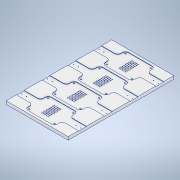
# Autodesk Inventor part: Tamale Assembly Plate
Saved by Autodesk Inventor 2022 (Build 260153000, 153)
## iProperties
Created: 2021-07-16
Part Number: Tamale Assembly Plate
Material: Aluminum 6061
Document SubType Name: Modeling
Designer: Caleb
Density: 2.7 g/cm^3
Appearance: Aluminum - Flat
Author: Caleb
Autodesk Inventor part; units mm, degrees
ref_plane "YZ Plane" through (0, 0, 0) normal (1, 0, 0) x (0, 1, 0)
ref_plane "XZ Plane" through (0, 0, 0) normal (0, 1, 0) x (-1, 0, 0)
ref_plane "XY Plane" through (0, 0, 0) normal (0, 0, 1) x (1, 0, 0)
sketch "Sketch1" plane through (0, 0, 0) normal (0, 1, 0) x (-1, 0, 0)
  line L0 (-63.5, 107.95) -> (63.5, 107.95)
  line L1 (63.5, 107.95) -> (63.5, -107.95)
  line L2 (63.5, -107.95) -> (-63.5, -107.95)
  line L3 (-63.5, -107.95) -> (-63.5, 107.95)
  line L4 (-63.5, 107.95) -> (63.5, -107.95) construction
  line L5 (63.5, 107.95) -> (-63.5, -107.95) construction
  point P0 (0, 0)
  dimension "d0" = 215.9
  dimension "d1" = 127
  constraints: 12 end point, 2 midpoint, 2 parallel, 1 horizontal, 1 perpendicular
  measures "d0" distance of L0.end L1.end
  measures "d1" distance of L1.end L2.end
extrude "Extrusion1" add sketch "Sketch1" along normal blind 6.35
sketch "Sketch2" plane through (0, 6.35, 0) normal (0, 1, 0) x (1, 0, 0)
  line L0 (23.8125, -102.87) -> (-23.8125, -102.87)
  line L1 (-30.1625, -96.52) -> (-30.1625, -93.345)
  line L2 (-23.8125, -55.245) -> (23.8125, -55.245)
  line L3 (30.1625, -93.345) -> (30.1625, -96.52)
  line L4 (30.1625, -102.87) -> (-30.1625, -55.245) construction
  line L5 (-30.1625, -102.87) -> (30.1625, -55.245) construction
  line L6 (-63.5, 107.95) -> (-63.5, -107.95) projected
  line L7 (-36.5125, -86.995) -> (-63.5, -86.995)
  line L8 (-63.5, -86.995) -> (-63.5, -71.12)
  line L9 (-63.5, -71.12) -> (-36.5125, -71.12)
  line L10 (63.5, -107.95) -> (63.5, 107.95) projected
  line L11 (36.5125, -71.12) -> (63.5, -71.12)
  line L12 (63.5, -71.12) -> (63.5, -86.995)
  line L13 (63.5, -86.995) -> (36.5125, -86.995)
  arc A0 (-30.1625, -96.52) -> (-23.8125, -102.87) centre (-23.8125, -96.52) ccw
  arc A1 (23.8125, -102.87) -> (30.1625, -96.52) centre (23.8125, -96.52) ccw
  arc A2 (-30.1625, -93.345) -> (-36.5125, -86.995) centre (-36.5125, -93.345) ccw
  arc A3 (36.5125, -86.995) -> (30.1625, -93.345) centre (36.5125, -93.345) ccw
  line L14 (-30.1625, -64.77) -> (-30.1625, -61.595)
  line L15 (30.1625, -64.77) -> (30.1625, -61.595)
  arc A4 (-36.5125, -71.12) -> (-30.1625, -64.77) centre (-36.5125, -64.77) ccw
  arc A5 (30.1625, -64.77) -> (36.5125, -71.12) centre (36.5125, -64.77) ccw
  arc A6 (30.1625, -61.595) -> (23.8125, -55.245) centre (23.8125, -61.595) ccw
  arc A7 (-23.8125, -55.245) -> (-30.1625, -61.595) centre (-23.8125, -61.595) ccw
  arc A8 (30.1625, -8.89) -> (23.8125, -2.54) centre (23.8125, -8.89) ccw
  line L16 (30.1625, -12.065) -> (30.1625, -8.89)
  line L17 (36.5125, -18.415) -> (63.5, -18.415)
  arc A9 (30.1625, -12.065) -> (36.5125, -18.415) centre (36.5125, -12.065) ccw
  line L18 (63.5, -18.415) -> (63.5, -34.29)
  line L19 (63.5, -34.29) -> (36.5125, -34.29)
  line L20 (-23.8125, -2.54) -> (23.8125, -2.54)
  line L21 (30.1625, -40.64) -> (30.1625, -43.815)
  arc A10 (23.8125, -50.165) -> (30.1625, -43.815) centre (23.8125, -43.815) ccw
  line L22 (-30.1625, -43.815) -> (-30.1625, -40.64)
  line L23 (23.8125, -50.165) -> (-23.8125, -50.165)
  line L24 (-30.1625, -50.165) -> (30.1625, -2.54) construction
  line L25 (30.1625, -50.165) -> (-30.1625, -2.54) construction
  arc A11 (36.5125, -34.29) -> (30.1625, -40.64) centre (36.5125, -40.64) ccw
  line L26 (-36.5125, -34.29) -> (-63.5, -34.29)
  line L27 (-63.5, -34.29) -> (-63.5, -18.415)
  line L28 (-63.5, -18.415) -> (-36.5125, -18.415)
  arc A12 (-23.8125, -2.54) -> (-30.1625, -8.89) centre (-23.8125, -8.89) ccw
  line L29 (-30.1625, -12.065) -> (-30.1625, -8.89)
  arc A13 (-36.5125, -18.415) -> (-30.1625, -12.065) centre (-36.5125, -12.065) ccw
  arc A14 (-30.1625, -43.815) -> (-23.8125, -50.165) centre (-23.8125, -43.815) ccw
  arc A15 (-30.1625, -40.64) -> (-36.5125, -34.29) centre (-36.5125, -40.64) ccw
  arc A16 (30.1625, 43.815) -> (23.8125, 50.165) centre (23.8125, 43.815) ccw
  line L30 (30.1625, 40.64) -> (30.1625, 43.815)
  line L31 (36.5125, 34.29) -> (63.5, 34.29)
  arc A17 (30.1625, 40.64) -> (36.5125, 34.29) centre (36.5125, 40.64) ccw
  line L32 (63.5, 34.29) -> (63.5, 18.415)
  line L33 (63.5, 18.415) -> (36.5125, 18.415)
  line L34 (-23.8125, 50.165) -> (23.8125, 50.165)
  line L35 (30.1625, 12.065) -> (30.1625, 8.89)
  arc A18 (23.8125, 2.54) -> (30.1625, 8.89) centre (23.8125, 8.89) ccw
  line L36 (-30.1625, 8.89) -> (-30.1625, 12.065)
  line L37 (23.8125, 2.54) -> (-23.8125, 2.54)
  line L38 (-30.1625, 2.54) -> (30.1625, 50.165) construction
  line L39 (30.1625, 2.54) -> (-30.1625, 50.165) construction
  arc A19 (36.5125, 18.415) -> (30.1625, 12.065) centre (36.5125, 12.065) ccw
  line L40 (-36.5125, 18.415) -> (-63.5, 18.415)
  line L41 (-63.5, 18.415) -> (-63.5, 34.29)
  line L42 (-63.5, 34.29) -> (-36.5125, 34.29)
  arc A20 (-23.8125, 50.165) -> (-30.1625, 43.815) centre (-23.8125, 43.815) ccw
  line L43 (-30.1625, 40.64) -> (-30.1625, 43.815)
  arc A21 (-36.5125, 34.29) -> (-30.1625, 40.64) centre (-36.5125, 40.64) ccw
  arc A22 (-30.1625, 8.89) -> (-23.8125, 2.54) centre (-23.8125, 8.89) ccw
  arc A23 (-30.1625, 12.065) -> (-36.5125, 18.415) centre (-36.5125, 12.065) ccw
  arc A24 (30.1625, 96.52) -> (23.8125, 102.87) centre (23.8125, 96.52) ccw
  line L44 (30.1625, 93.345) -> (30.1625, 96.52)
  line L45 (36.5125, 86.995) -> (63.5, 86.995)
  arc A25 (30.1625, 93.345) -> (36.5125, 86.995) centre (36.5125, 93.345) ccw
  line L46 (63.5, 86.995) -> (63.5, 71.12)
  line L47 (63.5, 71.12) -> (36.5125, 71.12)
  line L48 (-23.8125, 102.87) -> (23.8125, 102.87)
  line L49 (30.1625, 64.77) -> (30.1625, 61.595)
  arc A26 (23.8125, 55.245) -> (30.1625, 61.595) centre (23.8125, 61.595) ccw
  line L50 (-30.1625, 61.595) -> (-30.1625, 64.77)
  line L51 (23.8125, 55.245) -> (-23.8125, 55.245)
  line L52 (-30.1625, 55.245) -> (30.1625, 102.87) construction
  line L53 (30.1625, 55.245) -> (-30.1625, 102.87) construction
  arc A27 (36.5125, 71.12) -> (30.1625, 64.77) centre (36.5125, 64.77) ccw
  line L54 (-36.5125, 71.12) -> (-63.5, 71.12)
  line L55 (-63.5, 71.12) -> (-63.5, 86.995)
  line L56 (-63.5, 86.995) -> (-36.5125, 86.995)
  arc A28 (-23.8125, 102.87) -> (-30.1625, 96.52) centre (-23.8125, 96.52) ccw
  line L57 (-30.1625, 93.345) -> (-30.1625, 96.52)
  arc A29 (-36.5125, 86.995) -> (-30.1625, 93.345) centre (-36.5125, 93.345) ccw
  arc A30 (-30.1625, 61.595) -> (-23.8125, 55.245) centre (-23.8125, 61.595) ccw
  arc A31 (-30.1625, 64.77) -> (-36.5125, 71.12) centre (-36.5125, 64.77) ccw
  line L58 (-63.5, -107.95) -> (63.5, -107.95) projected
  point P0 (0, 0)
  point P1 (0, -79.0575)
  point P2 (30.1625, -71.12)
  point P3 (30.1625, -18.415)
  point P4 (0, -26.3525)
  point P5 (30.1625, 34.29)
  point P6 (0, 26.3525)
  point P7 (30.1625, 86.995)
  point P8 (0, 79.0575)
  point P9 (-63.5, 86.995)
  point P10 (-63.5, 71.12)
  point P11 (63.5, 71.12)
  point P12 (63.5, 86.995)
  point P13 (-63.5, 34.29)
  point P14 (-63.5, 18.415)
  point P15 (63.5, 18.415)
  point P16 (63.5, 34.29)
  point P17 (-63.5, -18.415)
  point P18 (-63.5, -34.29)
  point P19 (63.5, -34.29)
  point P20 (63.5, -18.415)
  point P21 (63.5, -71.12)
  point P22 (-63.5, -86.995)
  dimension "d4" = 60.325
  dimension "d5" = 47.625
  dimension "d6" = 15.875
  dimension "d7" = 6.35
  dimension "d8" = 6.35
  dimension "d9" = 15.875
  dimension "d10" = 15.875
  dimension "d11" = 15.875
  dimension "d14" = 52.705
  dimension "d19" = 5.08
  constraints: 112 end point, 64 point on circle, 54 point on line, 32 centre point, 16 tangent, 8 midpoint, 6 equal radius, 5 parallel, 3 horizontal, 3 perpendicular, 2 vertical, 168 other
  measures "d4" distance of L4.end L5.end
  measures "d5" distance of L5.start L4.end
  measures "d6" distance between parallel lines of L7 L9
  measures "d7" radius of A0
  measures "d8" radius of A4
  measures "d9" distance between parallel lines of L0 L7
  measures "d10" distance between parallel lines of L13 L0
  measures "d11" distance between parallel lines of L11 L13
  measures "d14" distance of L4.start L25.start
  measures "d19" distance between parallel lines of L58 L0
extrude "Extrusion2" cut sketch "Sketch2" against normal blind 0.863 contours L0 A0 L1 A2 L7 L6 L9 A4 L14 A7 L2 A6 L15 A5 L11 L10 L13 A3 L3 A1 | L19 A11 L21 A10 L23 A14 L22 A15 L26 L6 L28 A13 L29 A12 L20 A8 L16 A9 L17 L10 | L33 A19 L35 A18 L37 A22 L36 A23 L40 L6 L42 A21 L43 A20 L34 A16 L30 A17 L31 L10 | L47 A27 L49 A26 L51 A30 L50 A31 L54 L6 L56 A29 L57 A28 L48 A24 L44 A25 L45 L10
sketch "Sketch3" plane through (0, 5.487, 0) normal (0, 1, 0) x (1, 0, 0)
  line L0 (63.5, -71.12) -> (63.5, -86.995) projected
  line L1 (63.5, -86.995) -> (36.5125, -86.995) projected
  line L2 (36.5125, -71.12) -> (63.5, -71.12) projected
  line L3 (-63.5, -86.995) -> (-63.5, -71.12) projected
  point P0 (0, 0)
  point P1 (50.8, -79.0575)
  point P2 (-50.8, -79.0575)
  point P3 (-50.8, -26.3525)
  point P4 (50.8, -26.3525)
  point P5 (-50.8, 26.3525)
  point P6 (50.8, 26.3525)
  point P7 (-50.8, 79.0575)
  point P8 (50.8, 79.0575)
  point P9 (60.325, -79.0575)
  point P10 (-60.325, -79.0575)
  point P11 (60.325, -26.3525)
  point P12 (-60.325, -26.3525)
  point P13 (60.325, 26.3525)
  point P14 (-60.325, 26.3525)
  point P15 (60.325, 79.0575)
  point P16 (-60.325, 79.0575)
  dimension "d22" = 12.7
  dimension "d23" = 7.9375
  dimension "d25" = 12.7
  dimension "d28" = 52.705
  dimension "d40" = 3.175
  dimension "d41" = 3.175
  dimension "d44" = 52.705
  constraints: 3 horizontal alignment, 2 vertical, 12 other
  measures "d22" distance from line of L0 point (50.8, -79.057)
  measures "d23" distance from line of L1 point (50.8, -79.057)
  measures "d25" distance from line of L3 point (-50.8, -79.057)
  measures "d28" distance of point (-50.8, -79.057) point (-50.8, -26.352)
  measures "d40" distance from line of L0 point (60.325, -79.057)
  measures "d41" distance from line of L3 point (-60.325, -79.057)
  measures "d44" distance of point (60.325, -79.057) point (60.325, -26.352)
hole "Hole1" at (50.8, 5.487, 79.0575) at (-50.8, 5.487, 79.0575) at (-50.8, 5.487, 26.3525) at (50.8, 5.487, 26.3525) at (-50.8, 5.487, -26.3525) at (50.8, 5.487, -26.3525) at (-50.8, 5.487, -79.0575) at (50.8, 5.487, -79.0575) at (60.325, 5.487, 79.0575) at (60.325, 5.487, 26.3525) at (60.325, 5.487, -26.3525) at (60.325, 5.487, -79.0575) at (-60.325, 5.487, -79.0575) at (-60.325, 5.487, -26.3525) at (-60.325, 5.487, 26.3525) at (-60.325, 5.487, 79.0575) direction (0, -1, 0) diameter 1.0211 end through all thread size "00-96 NS" class "2B" standard "ANSI Unified Screw Threads"
sketch "Sketch4" plane through (0, 5.487, 0) normal (0, 1, 0) x (1, 0, 0)
  line L0 (23.8125, -102.87) -> (-23.8125, -102.87) projected
  line L1 (-30.1625, -64.77) -> (-30.1625, -61.595) projected
  point P0 (0, 0)
  point P1 (-25.8, -98.1575)
  point P2 (-25.8, -59.8575)
  point P3 (25.8, -59.8575)
  point P4 (25.8, -98.1575)
  point P5 (25.8, -7.1525)
  point P6 (-25.8, -7.1525)
  point P7 (-25.8, -45.4525)
  point P8 (25.8, -45.4525)
  point P9 (25.8, 45.5525)
  point P10 (-25.8, 45.5525)
  point P11 (-25.8, 7.2525)
  point P12 (25.8, 7.2525)
  point P13 (25.8, 98.2575)
  point P14 (-25.8, 98.2575)
  point P15 (-25.8, 59.9575)
  point P16 (25.8, 59.9575)
  dimension "d61" = 52.705
  constraints: 2 horizontal alignment, 2 vertical alignment, 1 vertical, 12 other
  measures "d61" distance of point (25.8, -59.857) point (25.8, -7.152)
hole "Hole2" at (-25.8, 5.487, 98.1575) at (-25.8, 5.487, 59.8575) at (25.8, 5.487, 59.8575) at (25.8, 5.487, 98.1575) at (25.8, 5.487, 7.1525) at (-25.8, 5.487, 7.1525) at (-25.8, 5.487, 45.4525) at (25.8, 5.487, 45.4525) at (25.8, 5.487, -45.5525) at (-25.8, 5.487, -45.5525) at (-25.8, 5.487, -7.2525) at (25.8, 5.487, -7.2525) at (25.8, 5.487, -98.2575) at (-25.8, 5.487, -98.2575) at (-25.8, 5.487, -59.9575) at (25.8, 5.487, -59.9575) direction (0, -1, 0) diameter 2.5 end through all
sketch "Sketch5" plane through (0, 5.487, 0) normal (0, 1, 0) x (1, 0, 0)
  line L0 (-23.8125, -55.245) -> (23.8125, -55.245) projected
  line L1 (23.8125, -102.87) -> (-23.8125, -102.87) projected
  line L2 (0, -79.0575) -> (0, -70.5908)
  line L3 (0, -70.5908) -> (9.1337, -70.5908)
  line L4 (0, -26.3525) -> (0, -17.8858)
  line L5 (0, -17.8858) -> (9.1337, -17.8858)
  line L6 (0, 26.3525) -> (0, 34.8192)
  line L7 (0, 34.8192) -> (9.1337, 34.8192)
  line L8 (0, 79.0575) -> (0, 87.5242)
  line L9 (0, 87.5242) -> (9.1337, 87.5242)
  point P0 (0, 0)
  point P1 (-6.35, -91.7575)
  point P2 (-6.35, -88.5825)
  point P3 (-6.35, -85.4075)
  point P4 (-6.35, -82.2325)
  point P5 (-6.35, -79.0575)
  point P6 (-6.35, -75.8825)
  point P7 (-6.35, -72.7075)
  point P8 (-6.35, -69.5325)
  point P9 (-6.35, -66.3575)
  point P10 (-3.175, -91.7575)
  point P11 (-3.175, -88.5825)
  point P12 (-3.175, -85.4075)
  point P13 (-3.175, -82.2325)
  point P14 (-3.175, -79.0575)
  point P15 (-3.175, -75.8825)
  point P16 (-3.175, -72.7075)
  point P17 (-3.175, -69.5325)
  point P18 (-3.175, -66.3575)
  point P19 (0, -91.7575)
  point P20 (0, -88.5825)
  point P21 (0, -85.4075)
  point P22 (0, -82.2325)
  point P23 (0, -79.0575)
  point P24 (0, -75.8825)
  point P25 (0, -72.7075)
  point P26 (0, -69.5325)
  point P27 (0, -66.3575)
  point P28 (3.175, -91.7575)
  point P29 (3.175, -88.5825)
  point P30 (3.175, -85.4075)
  point P31 (3.175, -82.2325)
  point P32 (3.175, -79.0575)
  point P33 (3.175, -75.8825)
  point P34 (3.175, -72.7075)
  point P35 (3.175, -69.5325)
  point P36 (3.175, -66.3575)
  point P37 (6.35, -91.7575)
  point P38 (6.35, -88.5825)
  point P39 (6.35, -85.4075)
  point P40 (6.35, -82.2325)
  point P41 (6.35, -79.0575)
  point P42 (6.35, -75.8825)
  point P43 (6.35, -72.7075)
  point P44 (6.35, -69.5325)
  point P45 (6.35, -66.3575)
  point P46 (6.35, -13.6525)
  point P47 (6.35, -16.8275)
  point P48 (6.35, -20.0025)
  point P49 (6.35, -23.1775)
  point P50 (6.35, -26.3525)
  point P51 (6.35, -29.5275)
  point P52 (6.35, -32.7025)
  point P53 (6.35, -35.8775)
  point P54 (6.35, -39.0525)
  point P55 (3.175, -13.6525)
  point P56 (3.175, -16.8275)
  point P57 (3.175, -20.0025)
  point P58 (3.175, -23.1775)
  point P59 (3.175, -26.3525)
  point P60 (3.175, -29.5275)
  point P61 (3.175, -32.7025)
  point P62 (3.175, -35.8775)
  point P63 (3.175, -39.0525)
  point P64 (0, -13.6525)
  point P65 (0, -16.8275)
  point P66 (0, -20.0025)
  point P67 (0, -23.1775)
  point P68 (0, -26.3525)
  point P69 (0, -29.5275)
  point P70 (0, -32.7025)
  point P71 (0, -35.8775)
  point P72 (0, -39.0525)
  point P73 (-3.175, -13.6525)
  point P74 (-3.175, -16.8275)
  point P75 (-3.175, -20.0025)
  point P76 (-3.175, -23.1775)
  point P77 (-3.175, -26.3525)
  point P78 (-3.175, -29.5275)
  point P79 (-3.175, -32.7025)
  point P80 (-3.175, -35.8775)
  point P81 (-3.175, -39.0525)
  point P82 (-6.35, -13.6525)
  point P83 (-6.35, -16.8275)
  point P84 (-6.35, -20.0025)
  point P85 (-6.35, -23.1775)
  point P86 (-6.35, -26.3525)
  point P87 (-6.35, -29.5275)
  point P88 (-6.35, -32.7025)
  point P89 (-6.35, -35.8775)
  point P90 (-6.35, -39.0525)
  point P91 (6.35, 39.0525)
  point P92 (6.35, 35.8775)
  point P93 (6.35, 32.7025)
  point P94 (6.35, 29.5275)
  point P95 (6.35, 26.3525)
  point P96 (6.35, 23.1775)
  point P97 (6.35, 20.0025)
  point P98 (6.35, 16.8275)
  point P99 (6.35, 13.6525)
  point P100 (3.175, 39.0525)
  point P101 (3.175, 35.8775)
  point P102 (3.175, 32.7025)
  point P103 (3.175, 29.5275)
  point P104 (3.175, 26.3525)
  point P105 (3.175, 23.1775)
  point P106 (3.175, 20.0025)
  point P107 (3.175, 16.8275)
  point P108 (3.175, 13.6525)
  point P109 (0, 39.0525)
  point P110 (0, 35.8775)
  point P111 (0, 32.7025)
  point P112 (0, 29.5275)
  point P113 (0, 26.3525)
  point P114 (0, 23.1775)
  point P115 (0, 20.0025)
  point P116 (0, 16.8275)
  point P117 (0, 13.6525)
  point P118 (-3.175, 39.0525)
  point P119 (-3.175, 35.8775)
  point P120 (-3.175, 32.7025)
  point P121 (-3.175, 29.5275)
  point P122 (-3.175, 26.3525)
  point P123 (-3.175, 23.1775)
  point P124 (-3.175, 20.0025)
  point P125 (-3.175, 16.8275)
  point P126 (-3.175, 13.6525)
  point P127 (-6.35, 39.0525)
  point P128 (-6.35, 35.8775)
  point P129 (-6.35, 32.7025)
  point P130 (-6.35, 29.5275)
  point P131 (-6.35, 26.3525)
  point P132 (-6.35, 23.1775)
  point P133 (-6.35, 20.0025)
  point P134 (-6.35, 16.8275)
  point P135 (-6.35, 13.6525)
  point P136 (6.35, 91.7575)
  point P137 (6.35, 88.5825)
  point P138 (6.35, 85.4075)
  point P139 (6.35, 82.2325)
  point P140 (6.35, 79.0575)
  point P141 (6.35, 75.8825)
  point P142 (6.35, 72.7075)
  point P143 (6.35, 69.5325)
  point P144 (6.35, 66.3575)
  point P145 (3.175, 91.7575)
  point P146 (3.175, 88.5825)
  point P147 (3.175, 85.4075)
  point P148 (3.175, 82.2325)
  point P149 (3.175, 79.0575)
  point P150 (3.175, 75.8825)
  point P151 (3.175, 72.7075)
  point P152 (3.175, 69.5325)
  point P153 (3.175, 66.3575)
  point P154 (0, 91.7575)
  point P155 (0, 88.5825)
  point P156 (0, 85.4075)
  point P157 (0, 82.2325)
  point P158 (0, 79.0575)
  point P159 (0, 75.8825)
  point P160 (0, 72.7075)
  point P161 (0, 69.5325)
  point P162 (0, 66.3575)
  point P163 (-3.175, 91.7575)
  point P164 (-3.175, 88.5825)
  point P165 (-3.175, 85.4075)
  point P166 (-3.175, 82.2325)
  point P167 (-3.175, 79.0575)
  point P168 (-3.175, 75.8825)
  point P169 (-3.175, 72.7075)
  point P170 (-3.175, 69.5325)
  point P171 (-3.175, 66.3575)
  point P172 (-6.35, 91.7575)
  point P173 (-6.35, 88.5825)
  point P174 (-6.35, 85.4075)
  point P175 (-6.35, 82.2325)
  point P176 (-6.35, 79.0575)
  point P177 (-6.35, 75.8825)
  point P178 (-6.35, 72.7075)
  point P179 (-6.35, 69.5325)
  point P180 (-6.35, 66.3575)
  dimension "d73" = 23.8125
  dimension "d75" = 12.7
  dimension "d76" = 6.35
  dimension "d79" = 3.175
  dimension "d82" = 3.175
  dimension "d87" = 52.705
  constraints: 16 end point, 3 vertical, 1 collinear, 1 horizontal, 1 perpendicular, 193 other
  measures "d73" distance from line of L0 L2.start
  measures "d75" vertical distance of point (-6.35, -91.757) L2.start
  measures "d76" horizontal distance of L2.start point (-6.35, -91.757)
  measures "d79" distance of point (-6.35, -91.757) point (-6.35, -88.582)
  measures "d82" distance of point (-6.35, -91.757) point (-3.175, -91.757)
  measures "d87" distance of L2.end L4.end
hole "Hole3" at (0, 5.487, 79.0575) at (-6.35, 5.487, 91.7575) at (-6.35, 5.487, 88.5825) at (-6.35, 5.487, 85.4075) at (-6.35, 5.487, 82.2325) at (-6.35, 5.487, 79.0575) at (-6.35, 5.487, 75.8825) at (-6.35, 5.487, 72.7075) at (-6.35, 5.487, 69.5325) at (-6.35, 5.487, 66.3575) at (-3.175, 5.487, 91.7575) at (-3.175, 5.487, 88.5825) at (-3.175, 5.487, 85.4075) at (-3.175, 5.487, 82.2325) at (-3.175, 5.487, 79.0575) at (-3.175, 5.487, 75.8825) at (-3.175, 5.487, 72.7075) at (-3.175, 5.487, 69.5325) at (-3.175, 5.487, 66.3575) at (0, 5.487, 91.7575) at (0, 5.487, 88.5825) at (0, 5.487, 85.4075) at (0, 5.487, 82.2325) at (0, 5.487, 75.8825) at (0, 5.487, 72.7075) at (0, 5.487, 69.5325) at (0, 5.487, 66.3575) at (3.175, 5.487, 91.7575) at (3.175, 5.487, 88.5825) at (3.175, 5.487, 85.4075) at (3.175, 5.487, 82.2325) at (3.175, 5.487, 79.0575) at (3.175, 5.487, 75.8825) at (3.175, 5.487, 72.7075) at (3.175, 5.487, 69.5325) at (3.175, 5.487, 66.3575) at (6.35, 5.487, 91.7575) at (6.35, 5.487, 88.5825) at (6.35, 5.487, 85.4075) at (6.35, 5.487, 82.2325) at (6.35, 5.487, 79.0575) at (6.35, 5.487, 75.8825) at (6.35, 5.487, 72.7075) at (6.35, 5.487, 69.5325) at (6.35, 5.487, 66.3575) at (0, 5.487, 26.3525) at (6.35, 5.487, 13.6525) at (6.35, 5.487, 16.8275) at (6.35, 5.487, 20.0025) at (6.35, 5.487, 23.1775) direction (0, -1, 0) diameter 1.5875 end through all and at (6.35, 5.487, 26.3525) (6.35, 5.487, 29.5275) (6.35, 5.487, 32.7025) (6.35, 5.487, 35.8775) (6.35, 5.487, 39.0525) (3.175, 5.487, 13.6525) (3.175, 5.487, 16.8275) (3.175, 5.487, 20.0025) (3.175, 5.487, 23.1775) (3.175, 5.487, 26.3525) (3.175, 5.487, 29.5275) (3.175, 5.487, 32.7025) (3.175, 5.487, 35.8775) (3.175, 5.487, 39.0525) (0, 5.487, 13.6525) (0, 5.487, 16.8275) (0, 5.487, 20.0025) (0, 5.487, 23.1775) (0, 5.487, 29.5275) (0, 5.487, 32.7025) (0, 5.487, 35.8775) (0, 5.487, 39.0525) (-3.175, 5.487, 13.6525) (-3.175, 5.487, 16.8275) (-3.175, 5.487, 20.0025) (-3.175, 5.487, 23.1775) (-3.175, 5.487, 26.3525) (-3.175, 5.487, 29.5275) (-3.175, 5.487, 32.7025) (-3.175, 5.487, 35.8775) (-3.175, 5.487, 39.0525) (-6.35, 5.487, 13.6525) (-6.35, 5.487, 16.8275) (-6.35, 5.487, 20.0025) (-6.35, 5.487, 23.1775) (-6.35, 5.487, 26.3525) (-6.35, 5.487, 29.5275) (-6.35, 5.487, 32.7025) (-6.35, 5.487, 35.8775) (-6.35, 5.487, 39.0525) (0, 5.487, -26.3525) (6.35, 5.487, -39.0525) (6.35, 5.487, -35.8775) (6.35, 5.487, -32.7025) (6.35, 5.487, -29.5275) (6.35, 5.487, -26.3525) (6.35, 5.487, -23.1775) (6.35, 5.487, -20.0025) (6.35, 5.487, -16.8275) (6.35, 5.487, -13.6525) (3.175, 5.487, -39.0525) (3.175, 5.487, -35.8775) (3.175, 5.487, -32.7025) (3.175, 5.487, -29.5275) (3.175, 5.487, -26.3525) (3.175, 5.487, -23.1775) (3.175, 5.487, -20.0025) (3.175, 5.487, -16.8275) (3.175, 5.487, -13.6525) (0, 5.487, -39.0525) (0, 5.487, -35.8775) (0, 5.487, -32.7025) (0, 5.487, -29.5275) (0, 5.487, -23.1775) (0, 5.487, -20.0025) (0, 5.487, -16.8275) (0, 5.487, -13.6525) (-3.175, 5.487, -39.0525) (-3.175, 5.487, -35.8775) (-3.175, 5.487, -32.7025) (-3.175, 5.487, -29.5275) (-3.175, 5.487, -26.3525) (-3.175, 5.487, -23.1775) (-3.175, 5.487, -20.0025) (-3.175, 5.487, -16.8275) (-3.175, 5.487, -13.6525) (-6.35, 5.487, -39.0525) (-6.35, 5.487, -35.8775) (-6.35, 5.487, -32.7025) (-6.35, 5.487, -29.5275) (-6.35, 5.487, -26.3525) (-6.35, 5.487, -23.1775) (-6.35, 5.487, -20.0025) (-6.35, 5.487, -16.8275) (-6.35, 5.487, -13.6525) (0, 5.487, -79.0575) (6.35, 5.487, -91.7575) (6.35, 5.487, -88.5825) (6.35, 5.487, -85.4075) (6.35, 5.487, -82.2325) (6.35, 5.487, -79.0575) (6.35, 5.487, -75.8825) (6.35, 5.487, -72.7075) (6.35, 5.487, -69.5325) (6.35, 5.487, -66.3575) (3.175, 5.487, -91.7575) (3.175, 5.487, -88.5825) (3.175, 5.487, -85.4075) (3.175, 5.487, -82.2325) (3.175, 5.487, -79.0575) (3.175, 5.487, -75.8825) (3.175, 5.487, -72.7075) (3.175, 5.487, -69.5325) (3.175, 5.487, -66.3575) (0, 5.487, -91.7575) (0, 5.487, -88.5825) (0, 5.487, -85.4075) (0, 5.487, -82.2325) (0, 5.487, -75.8825) (0, 5.487, -72.7075) (0, 5.487, -69.5325) (0, 5.487, -66.3575) (-3.175, 5.487, -91.7575) (-3.175, 5.487, -88.5825) (-3.175, 5.487, -85.4075) (-3.175, 5.487, -82.2325) (-3.175, 5.487, -79.0575) (-3.175, 5.487, -75.8825) (-3.175, 5.487, -72.7075) (-3.175, 5.487, -69.5325) (-3.175, 5.487, -66.3575) (-6.35, 5.487, -91.7575) (-6.35, 5.487, -88.5825) (-6.35, 5.487, -85.4075) (-6.35, 5.487, -82.2325) (-6.35, 5.487, -79.0575) (-6.35, 5.487, -75.8825) (-6.35, 5.487, -72.7075) (-6.35, 5.487, -69.5325) (-6.35, 5.487, -66.3575)
body "Solid1"
